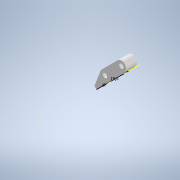
# Autodesk Inventor part: laser_krepl
Saved by Autodesk Inventor 2022 (Build 260153000, 153)
## iProperties
Created: 2023-01-26
Part Number: laser_krepl
Material: Типовые
Document SubType Name: Modeling
Designer: akapu
Density: 1 g/cm^3
Appearance: По умолчанию
Author: akapu
Autodesk Inventor part; units mm, degrees
ref_plane "YZ Plane" through (0, 0, 0) normal (1, 0, 0) x (0, 1, 0)
ref_plane "XZ Plane" through (0, 0, 0) normal (0, 1, 0) x (-1, 0, 0)
ref_plane "XY Plane" through (0, 0, 0) normal (0, 0, 1) x (1, 0, 0)
sketch "Эскиз1" plane through (0, 0, 0) normal (0, 0, 1) x (1, 0, 0)
  line L0 (153.1973, 25.2896) -> (151.2527, 27.2341) projected
  line L1 (153.9044, 25.9967) -> (151.9598, 27.9412) projected
  line L2 (135.5196, 42.9673) -> (137.4641, 41.0227) projected
  line L3 (136.2267, 43.6744) -> (138.1712, 41.7298) projected
  line L4 (138.7016, 39.7853) -> (150.0153, 28.4716) projected
  line L5 (150.7224, 29.1787) -> (150.0153, 28.4716) projected
  line L6 (139.4087, 40.4924) -> (150.7224, 29.1787) projected
  line L7 (139.4087, 40.4924) -> (138.7016, 39.7853) projected
  line L8 (137.4641, 41.0227) -> (138.7016, 39.7853) projected
  line L9 (138.1712, 41.7298) -> (139.4087, 40.4924) projected
  line L10 (151.9598, 27.9412) -> (150.7224, 29.1787) projected
  line L11 (151.2527, 27.2341) -> (150.0153, 28.4716) projected
  line L12 (148.6011, 28.4716) -> (146.4797, 30.5929) projected
  line L13 (143.2978, 33.7749) -> (141.8836, 35.1891) projected
  line L14 (140.7168, 37.0629) -> (140.1158, 37.664) projected
  line L15 (139.6562, 38.1236) -> (139.0551, 38.7246) projected
  line L16 (144.1817, 37.1336) -> (147.3636, 33.9517) projected
  line L17 (145.2883, 32.0672) -> (144.6872, 32.6683) projected
  line L18 (144.0933, 33.2622) -> (143.4922, 33.8633) projected
  line L19 (146.1262, 31.6536) -> (144.8534, 32.9263) projected
  line L20 (148.0354, 29.3201) -> (146.904, 30.4515) projected
  line L21 (136.2267, -54.0744) -> (138.1712, -52.1298) projected
  line L22 (135.5196, -53.3673) -> (137.4641, -51.4227) projected
  line L23 (140.4767, -49.8244) -> (139.7696, -49.1173)
  line L24 (137.4641, -51.4227) -> (138.7016, -50.1853) projected
  line L25 (138.1712, -52.1298) -> (139.4087, -50.8924) projected
  line L26 (150.0153, -38.8716) -> (138.7016, -50.1853) projected
  line L27 (139.4087, -50.8924) -> (138.7016, -50.1853) projected
  line L28 (150.7224, -39.5787) -> (139.4087, -50.8924) projected
  line L29 (150.7224, -39.5787) -> (150.0153, -38.8716) projected
  line L30 (151.2527, -37.6341) -> (150.0153, -38.8716) projected
  line L31 (151.9598, -38.3412) -> (150.7224, -39.5787) projected
  line L32 (153.9044, -36.3967) -> (151.9598, -38.3412) projected
  line L33 (153.1973, -35.6896) -> (151.2527, -37.6341) projected
  line L34 (158.1544, -32.1467) -> (157.4473, -31.4396)
  line L35 (147.3636, -44.3517) -> (144.1817, -47.5336) projected
  line L36 (138.7016, -48.7711) -> (140.8229, -46.6497) projected
  line L37 (139.5501, -48.2054) -> (140.6815, -47.074) projected
  line L38 (141.8836, -46.2962) -> (143.1563, -45.0234) projected
  line L39 (142.2972, -45.4583) -> (142.8983, -44.8572) projected
  line L40 (143.4922, -44.2633) -> (144.0933, -43.6622) projected
  line L41 (144.6872, -43.0683) -> (145.2883, -42.4672) projected
  line L42 (144.0049, -43.4678) -> (145.4191, -42.0536) projected
  line L43 (147.2929, -40.8868) -> (147.894, -40.2858) projected
  line L44 (148.3536, -39.8262) -> (148.9546, -39.2251) projected
  ellipse E0 centre (88.75, 20.1064) end of major axis (88.75, -5.3184) minor radius 3 (89.0392, -5.2) -> (90.4149, -1.0438) ccw projected
  ellipse E1 centre (88.75, -30.5064) end of major axis (88.75, -5.0816) minor radius 3 (90.4149, -9.3562) -> (89.0392, -5.2) ccw projected
  line L45 (117.53, -9.3562) -> (90.4149, -9.3562) projected
  line L46 (117.53, -13.227) -> (117.53, -9.3562) projected
  line L47 (139.4449, -26.6135) -> (117.53, -13.227) projected
  arc A0 (139.4449, -26.6135) -> (145.2751, -24.6051) centre (141.53, -23.2) ccw projected
  line L48 (150.53, -10.5988) -> (145.2751, -24.6051) projected
  line L49 (150.53, -10.5988) -> (150.53, 0.6151) projected
  line L50 (145.2608, 14.2426) -> (150.53, 0.6151) projected
  arc A1 (145.2608, 14.2426) -> (139.4449, 16.2135) centre (141.53, 12.8) ccw projected
  line L51 (117.53, 2.827) -> (139.4449, 16.2135) projected
  line L52 (117.53, -1.0438) -> (117.53, 2.827) projected
  line L53 (90.4149, -1.0438) -> (117.53, -1.0438) projected
  circle A2 centre (141.53, 12.8) radius 1.6 projected
  circle A3 centre (141.53, -23.2) radius 1.6 projected
  circle A4 centre (141.53, -41.7) radius 13.463
  line L54 (141.53, -41.7) -> (145.53, -41.7) construction
  line L55 (144.3584, -44.5284) -> (153.4482, -35.4383)
  line L56 (153.4482, -35.4383) -> (135.2688, -53.6185)
  line L57 (135.2688, -53.6185) -> (134.3589, -52.7086)
  line L58 (135.2688, -53.6185) -> (132.4403, -50.7901)
  circle A5 centre (141.5299, -41.7001) radius 3.5
  circle A6 centre (141.5299, -41.7001) radius 1.6
  line L59 (153.4482, -35.4383) -> (150.6197, -32.6099)
  line L60 (144.3584, -44.5284) -> (141.5299, -41.7001)
  line L61 (150.6197, -32.6099) -> (132.4403, -50.7901)
  line L62 (150.6197, -32.6099) -> (153.4482, -29.7813)
  circle A7 centre (153.4482, -29.7813) radius 1.6
  circle A8 centre (153.4482, -29.7813) radius 3.5
  line L63 (153.4482, -35.4383) -> (156.1979, -31.9467)
  line L64 (150.9733, -27.3065) -> (139.0551, -39.2252)
  line L65 (133.8546, -52.2043) -> (138.2526, -40.4715)
  point P0 (0, 0)
  point P1 (132.4401, -45.8401)
  point P2 (134.3589, -52.7086)
  point P3 (135.5198, -53.3675)
  point P4 (144.3584, -44.5284)
  point P5 (139.0551, -44.175)
  point P6 (144.3584, -44.5284)
  dimension "d9" = 18.5
  dimension "d19" = 4
  dimension "d28" = 7
  dimension "d29" = 3.2
  dimension "d32" = 4
  dimension "d33" = 4
  dimension "d34" = 90
  dimension "d35" = 3.2
  dimension "d36" = 7
  constraints: 26 end point, 6 point on circle, 5 centre point, 4 coincident, 3 point on line, 3 tangent, 2 perpendicular, 1 horizontal, 1 midpoint, 9 other
  measures "d9" distance of A3.centre L54.start
  measures "d19" distance of L56.end L58.end
  measures "d28" diameter of A5
  measures "d29" diameter of A6
  measures "d32" distance of L55.end L59.end
  measures "d33" distance of L55.start L60.end
  measures "d34" angle of L59 L55
  measures "d35" diameter of A7
  measures "d36" diameter of A8
extrude "Выдавливание1" add sketch "Эскиз1" against normal blind 12 contours L57 L58 L65 L61 A5 L60 L26 L24 L22 L56 | L64 A8 A4 | A4 A8 L62 L61 A5 L64 | A8 A4 | A4 L62 A8 | A5 L61 A6 | L59 L62 A8 A4 | L55 L33 L30 L26 L60 A5 L61 L59 | A4 A8 L63 | A4 A8 L62 | A5 L61 L65 | A5 L60 A6 L61 | L61 A6 L60 A5
chamfer "Фаска1" distance 1 angle 45 2 edges at (139.9299, -41.7001, -12) (151.8482, -29.7813, -12)
sketch "Эскиз2" plane through (135.2688, -53.6185, 0) normal (0.7071227, -0.7070909, 0) x (0, 0, -1)
  line L0 (0, 11.255) -> (0, 14.455) projected
  line L1 (11, 14.455) -> (11, 11.255) projected
  line L2 (11, 31.3103) -> (11, 28.1103) projected
  line L3 (0, 28.1103) -> (0, 31.3103) projected
  line L4 (11, 31.3103) -> (11, 28.1103) projected
  line L5 (0, 28.1103) -> (0, 31.3103) projected
  line L6 (0, 31.3103) -> (12, 31.3103)
  line L7 (12, 27.1103) -> (12, 32.3103) projected
  line L8 (0, 28.1103) -> (8, 28.1103)
  line L9 (0, 11.255) -> (0, 14.455) projected
  line L10 (0, 14.455) -> (12, 14.455)
  line L11 (12, 10.255) -> (12, 15.455) projected
  line L12 (0, 11.255) -> (8, 11.255)
  line L13 (0, 0) -> (6, 0)
  line L14 (0, 0) -> (12, 0) projected
  line L15 (6, 0) -> (6, 33.2103)
  line L16 (0, 33.2103) -> (12, 33.2103) projected
  line L17 (6, 0) -> (6, 4.305)
  line L18 (6, 4.305) -> (6, 23.805)
  circle A0 centre (6, 23.805) radius 1.6
  circle A1 centre (6, 4.305) radius 1.6
  circle A2 centre (6, 23.805) radius 4.3053
  circle A3 centre (6, 4.305) radius 4.305
  point P0 (0, -57.7325)
  dimension "d40" = 6
  dimension "d41" = 4.305
  dimension "d42" = 19.5
  dimension "d43" = 3.2
  dimension "d44" = 3.2
  constraints: 16 end point, 4 coincident, 4 horizontal, 4 point on line, 3 centre point, 2 midpoint, 1 perpendicular, 1 vertical alignment, 2 other
  measures "d40" distance of L13.start L13.end
  measures "d41" distance of L13.end L17.end
  measures "d42" distance of L17.end L18.end
  measures "d43" diameter of A0
  measures "d44" diameter of A1
extrude "Выдавливание2" cut sketch "Эскиз2" against normal blind 10 contours A0 L15 | L15 A0 | A1 L15 | L15 A1
chamfer "Фаска2" distance 3.5 angle 45 4 edges at (135.3943, -53.493, -12) (136.492, -52.3951, -12) (140.9113, -47.9756, -12) (148.9033, -39.9833, -12)
sketch "Эскиз3" plane through (150.9733, -27.3065, -12) normal (-0.7071227, 0.7070909, 0) x (0, 0, 1)
  circle A0 centre (6, -5.9053) radius 1.6 projected
  line L0 (6, -5.9053) -> (8.7, -5.9053)
  line L1 (12, 0) -> (12, -16.8552) projected
  line L2 (8.7, -7.4641) -> (6, -9.023)
  line L3 (6, -9.023) -> (3.3, -7.4641)
  line L4 (3.3, -7.4641) -> (3.3, -4.3464)
  line L5 (3.3, -4.3464) -> (6, -2.7876)
  line L6 (6, -2.7876) -> (8.7, -4.3464)
  line L7 (8.7, -4.3464) -> (8.7, -7.4641)
  point P0 (12, -87.4428)
  dimension "d50" = 2.7
  constraints: 14 end point, 1 coincident, 1 midpoint, 1 perpendicular, 13 other
  measures "d50" distance of L0.start L0.end
extrude "Выдавливание3" cut sketch "Эскиз3" against normal blind 1.5
sketch "Эскиз4" plane through (150.9733, -27.3065, -12) normal (-0.7071227, 0.7070909, 0) x (0, 0, 1)
  circle A0 centre (6, -25.4053) radius 1.6 projected
  line L0 (6, -25.4053) -> (8.7, -25.4053)
  line L1 (12, -29.7103) -> (12, -4.0002) projected
  line L2 (8.7, -26.9641) -> (6, -28.523)
  line L3 (6, -28.523) -> (3.3, -26.9641)
  line L4 (3.3, -26.9641) -> (3.3, -23.8464)
  line L5 (3.3, -23.8464) -> (6, -22.2876)
  line L6 (6, -22.2876) -> (8.7, -23.8464)
  line L7 (8.7, -23.8464) -> (8.7, -26.9641)
  point P0 (12, -87.4428)
  dimension "d53" = 2.7
  constraints: 14 end point, 1 coincident, 1 midpoint, 1 perpendicular, 13 other
  measures "d53" distance of L0.start L0.end
extrude "Выдавливание4" cut sketch "Эскиз4" against normal blind 5
